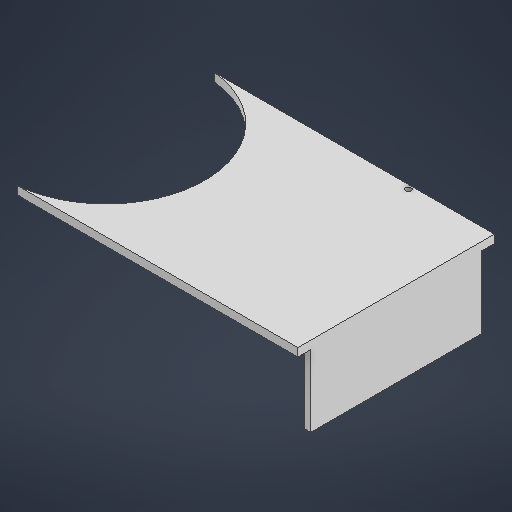
# Autodesk Inventor part: TAMPA_BASE
Saved by Autodesk Inventor 2027.1 (Build 311270010, 270A)
## iProperties
Created: 2026-08-16
Part Number: TAMPA_BASE
Material: Genérico
Document SubType Name: Modeling
Designer: Evellyn
Density: 1 g/cm^3
Appearance: Padrão
Author: Evellyn
Autodesk Inventor part; units mm, degrees
ref_plane "YZ Plane" through (0, 0, 0) normal (1, 0, 0) x (0, 1, 0)
ref_plane "XZ Plane" through (0, 0, 0) normal (0, 1, 0) x (-1, 0, 0)
ref_plane "XY Plane" through (0, 0, 0) normal (0, 0, 1) x (1, 0, 0)
sketch "Esboço1" plane through (0, 0, 0) normal (0, 1, 0) x (-1, 0, 0)
  line L0 (-70.859, -48) -> (70.859, -48)
  line L1 (70.859, 48) -> (-70.859, 48)
  line L2 (-70.859, 48) -> (-70.859, -48)
  line L3 (-70.859, -48) -> (70.859, 48) construction
  line L4 (70.859, -48) -> (-70.859, 48) construction
  arc A0 (66.1187, 48) -> (66.1187, -48) centre (70.859, 0) ccw
  circle A1 centre (-30.859, -46) radius 1.35
  point P0 (0, 0)
  dimension "d3" = 2.7
  dimension "d4" = 2
  dimension "d5" = 40
  constraints: 10 end point, 2 centre point, 2 midpoint, 2 point on circle, 2 point on line, 1 horizontal, 1 parallel
  measures "d3" diameter of A1
  measures "d4" distance from line of L0 A1.centre
  measures "d5" distance from line of L2 A1.centre
extrude "Extrusão1" add sketch "Esboço1" along normal blind 4
sketch "Esboço2" plane through (0, 0, 0) normal (0, -1, 0) x (1, 0, 0)
  line L0 (-66.1187, 48) -> (70.859, 48) projected
  line L1 (70.859, -48) -> (-66.1187, -48) projected
  line L2 (70.859, 48) -> (67.859, 48)
  line L3 (67.859, 48) -> (67.859, -48)
  line L4 (67.859, -48) -> (70.859, -48)
  line L5 (70.859, -48) -> (70.859, 48)
  line L6 (67.859, -41.75) -> (70.859, -41.75)
  line L7 (70.859, -41.75) -> (70.859, 41.75)
  line L8 (70.859, 41.75) -> (67.859, 41.75)
  line L9 (67.859, 41.75) -> (67.859, -41.75)
  line L10 (67.859, -41.75) -> (70.859, 41.75) construction
  line L11 (70.859, -41.75) -> (67.859, 41.75) construction
  point P0 (0, 0)
  point P1 (69.359, 0)
  dimension "d8" = 3
  dimension "d9" = 3
  dimension "d10" = 83.5
  constraints: 20 end point, 4 parallel, 2 horizontal, 2 midpoint, 2 perpendicular, 1 point on line
  measures "d8" distance of L4.end L3.end
  measures "d9" distance of L8.end L7.end
  measures "d10" distance of L7.end L6.end
extrude "Extrusão2" add sketch "Esboço2" along normal blind 35 contours L8 L5 L6 L3
